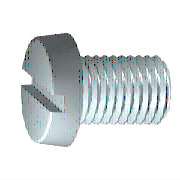
# Autodesk Inventor part: ISO 1207 - M4 x 14
Saved by Autodesk Inventor 2025.2 (Build 292293000, 293)
## iProperties
Created: 2024-01-20
Part Number: ISO 1207 - M4 x 14
Material: Stainless Steel, 440C
Description: Slotted cheese head screws - Product grade A
Document SubType Name: Modeling
Standard: ISO 1207
Designer: Kacper Mik
Standard Revision: Third edition 2011-08-01
Standards Organization: ISO
Language: en-US
Size Designation: M4 x 14
Categories: <MemberInstance><Categories><Category DisplayName="Fasteners" InternalName="e4da775c-781d-43d5-af7c-5136215cf5a6" Mnemonic="FSTN"><Category DisplayName="Bolts" InternalName="536e6df0-f778-49ac-b2f2-25c71d2aa0b2" Mnemonic="SCRW"><CategoryParameter DisplayName="Nominal Diameter Designation" InternalName="03caf894-eafd-4c09-a035-916ac084b87b" Mnemonic="nomdiadesig"/><CategoryParameter DisplayName="Nominal Length" InternalName="238ecbaf-3e6c-45dd-aa95-4068c8e0fd02" Mnemonic="nomlen"/><CategoryParameter DisplayName="Thread Designation" InternalName="586d5e89-370a-4089-914f-0110033585c7" Mnemonic="thrdesign"/><CategoryParameter DisplayName="Thread Series Designation" InternalName="87c5849c-b3a5-4c3e-9c9b-2feecef9be86" Mnemonic="thrserdsgn"/><CategoryParameter DisplayName="Nominal Diameter" InternalName="8bbe3f8e-44cf-40a9-a251-3a6edc8168d6" Mnemonic="nomdia"/><CategoryParameter DisplayName="Thread Type" InternalName="b4bbb7bc-d6aa-4c9f-a9a9-4152b9f6fe49" Mnemonic="thrtype"/><CategoryParameter DisplayName="Thread Pitch" InternalName="bb82302e-82d8-4176-8fc1-c5d7bb17d5ad" Mnemonic="pitch1"/><CategoryParameter DisplayName="Threads per Unit" InternalName="bdc6e7d2-ffd0-4d9c-a173-16b95ebb912d" Mnemonic="thrperunit1"/><CategoryParameter DisplayName="Thread Class" InternalName="ebc0d23b-2cc6-4d2a-b376-d52aae53bab6" Mnemonic="thrclss"/><Category DisplayName="Socket Head" InternalName="55e06bf3-7e58-486c-bbdc-745fcc60664d" Mnemonic="CLSCRW"><CategoryParameter DisplayName="Shank Diameter" InternalName="179dbae3-102f-48bb-85fe-1e3ecd34f7cc" Mnemonic="grpdia"/><CategoryParameter DisplayName="Thread Length" InternalName="3268731d-5f9a-4750-8b01-4a959c46fbf2" Mnemonic="thrlen"/><CategoryParameter DisplayName="Head Diameter" InternalName="46177176-dbdd-4a1b-aefd-4c60c45016af" Mnemonic="headdia"/><CategoryParameter DisplayName="Grip Length" InternalName="52eab69f-422f-4795-9995-175a1b827e67" Mnemonic="grplen"/><CategoryParameter DisplayName="Type" InternalName="59a7e495-7a0c-4a5c-bdfd-c090c5f6e2db" Mnemonic="type"/><CategoryParameter DisplayName="Head Height" InternalName="99c92c4c-4a02-4ebe-9e64-948fb169e19e" Mnemonic="headh"/></Category></Category></Category><Category DisplayName="DataType" InternalName="23b78d0f-2648-40c6-8793-ca6db495c9e8" Mnemonic="DATATYPE"><CategoryParameter DisplayName="DisplayName" InternalName="05415f3d-3907-474b-a020-eb9d644f4cf3" Mnemonic="DISPLAYNAME"/><CategoryParameter DisplayName="Standard" InternalName="0c0a119c-1e12-4c84-803f-101930972f5e" Mnemonic="STANDARD"/><CategoryParameter DisplayName="Description" InternalName="13903e3d-64b1-4950-80da-f627842ea37f" Mnemonic="DESCRIPTION"/><CategoryParameter DisplayName="Designation" InternalName="2675968c-4ce5-49e0-a4f5-552d29089031" Mnemonic="DESIGNATION"/><CategoryParameter DisplayName="Default Row" InternalName="2af9ec52-faaa-4026-b378-f9fa4afca842" Mnemonic="DEFAULTROW"/><CategoryParameter DisplayName="Folder Name" InternalName="3f06958e-8713-4116-9be7-ed6184ecc97b" Mnemonic="FOLDERNAME"/><CategoryParameter DisplayName="Revision Guid" InternalName="45a75005-10b1-4dfc-8d6d-dfe629f0b93c" Mnemonic="REVISIONGUID"/><CategoryParameter DisplayName="FileName" InternalName="8b46a4cc-9585-4fed-90c3-899f57e09a73" Mnemonic="FILENAME"/><CategoryParameter DisplayName="StdsOrg" InternalName="8f5914e1-4693-403f-8ab5-d37768198c9d" Mnemonic="STDSORG"/><CategoryParameter DisplayName="Family Version" InternalName="914462f6-6e19-4b14-ba84-155b9680b1d0" Mnemonic="FAMILYREVISION"/><CategoryParameter DisplayName="Standard Revision" InternalName="91d5a463-65c2-4fde-b823-3b7fea5e8e17" Mnemonic="STANDARDREVISION"/><CategoryParameter DisplayName="Member Revision" InternalName="a65d44b9-392f-4f4f-857b-e4b3d54996fe" Mnemonic="MEMBERREVISION"/><CategoryParameter DisplayName="ClipFormat" InternalName="bc51e27b-3422-4e78-93ef-cec197ddf230" Mnemonic="CLIPFORMAT"/><CategoryParameter DisplayName="Manufacturer" InternalName="cd6c7a72-a28a-4e50-99a9-2c7f4e13e5ad" Mnemonic="MANUFACTURER"/><CategoryParameter DisplayName="InternalName" InternalName="cf1d0246-76d9-4b4a-8305-fa0409afb5c1" Mnemonic="INTERNALNAME"/><CategoryParameter DisplayName="IsMetric" InternalName="e2385c5b-1ea4-4823-96a8-8de651266ec3" Mnemonic="ISMETRIC"/><Category DisplayName="Part" InternalName="c0e0b642-3bcb-4cc8-9e80-f96d35c4afa4" Mnemonic="PART"><CategoryParameter DisplayName="Part Number" InternalName="016b6077-bfbe-49bd-92c9-d8d59c39c941" Mnemonic="PARTNUMBER"/><CategoryParameter DisplayName="Stock Number" InternalName="4dba7c1c-e26c-444e-836c-b08b433409a8" Mnemonic="STOCKNUMBER"/><CategoryParameter DisplayName="Material Key" InternalName="5c9a8adb-dd2b-4535-b97f-0a94a95fe41f" Mnemonic="MATERIALKEY"/><CategoryParameter DisplayName="Material" InternalName="818a152a-d3c3-49ca-80ee-df7d91421b8e" Mnemonic="MATERIAL"/></Category></Category><Category DisplayName="Legacy Map DA" InternalName="924fff40-ddd0-4eff-ad42-30e3774ef79e" Mnemonic="LEGACYMAPDA"><CategoryParameter DisplayName="DACookie" InternalName="316934ee-8fe1-4c7a-9c36-f2d79e1add1a" Mnemonic="DACOOKIE"/></Category><Category DisplayName="LegacyMap" InternalName="cd87c42b-3e48-431e-b5c0-1cbeb14dfe77" Mnemonic="LEGACYMAP"><CategoryParameter DisplayName="unique DA member ID" InternalName="0918ad47-427f-4fed-ae26-24c81c58f590" Mnemonic="DACOOKIE"/><CategoryParameter DisplayName="Merge11 ID" InternalName="0ee8fb18-e2ed-4f39-96f6-1f4b5f50aa71" Mnemonic="MERGE11"/><CategoryParameter DisplayName="unique CC member ID" InternalName="5193edd4-b2b0-4ab4-9d54-de900eee34e0" Mnemonic="CCCOOKIE"/><CategoryParameter DisplayName="Split ID" InternalName="72b5c83c-be7f-45c4-ae51-9160ea6deb26" Mnemonic="SPLIT"/><CategoryParameter DisplayName="MemberID" InternalName="8e5e0294-fc51-4c8f-b3d7-003dc5ed94f6" Mnemonic="MEMBERID"/><CategoryParameter DisplayName="CatalogName" InternalName="d99d1e27-aa94-4de2-af4c-c348882a6f4f" Mnemonic="CATALOGNAME"/><CategoryParameter DisplayName="FamilyNumber" InternalName="e705e1f4-09cb-413e-91f9-551b4188271e" Mnemonic="FAMILYNUMBER"/></Category></Categories><FamilyTemplate Id="si0146"><FamilyTemplateParameters><FamilyTemplateParameter ObjectType="kUserParameterObject" ValueType="xs:double" Id="1" ObjectReferenceKey="GUL"/><FamilyTemplateParameter ObjectType="kUserParameterObject" ValueType="xs:double" Id="2" ObjectReferenceKey="SPD"/><FamilyTemplateParameter ObjectType="kUserParameterObject" ValueType="xs:double" Id="3" ObjectReferenceKey="NLG"/><FamilyTemplateParameter ObjectType="kUserParameterObject" ValueType="xs:double" Id="4" ObjectReferenceKey="KOD"/><FamilyTemplateParameter ObjectType="kUserParameterObject" ValueType="xs:double" Id="5" ObjectReferenceKey="SBR"/><FamilyTemplateParameter ObjectType="kUserParameterObject" ValueType="xs:double" Id="6" ObjectReferenceKey="PTC"/><FamilyTemplateParameter ObjectType="kUserParameterObject" ValueType="xs:double" Id="7" ObjectReferenceKey="GEL"/><FamilyTemplateParameter ObjectType="kUserParameterObject" ValueType="xs:double" Id="8" ObjectReferenceKey="THREADDIA"/><FamilyTemplateParameter ObjectType="kUserParameterObject" ValueType="xs:double" Id="9" ObjectReferenceKey="TOA"/><FamilyTemplateParameter ObjectType="kUserParameterObject" ValueType="xs:double" Id="10" ObjectReferenceKey="BDM"/><FamilyTemplateParameter ObjectType="kUserParameterObject" ValueType="xs:double" Id="11" ObjectReferenceKey="RR"/><FamilyTemplateParameter ObjectType="kUserParameterObject" ValueType="xs:double" Id="12" ObjectReferenceKey="STI"/><FamilyTemplateParameter ObjectType="kUserParameterObject" ValueType="xs:double" Id="13" ObjectReferenceKey="TPU"/><FamilyTemplateParameter ObjectType="kUserParameterObject" ValueType="xs:double" Id="14" ObjectReferenceKey="KOH"/><FamilyTemplateParameter ObjectType="kUserParameterObject" ValueType="xs:double" Id="15" ObjectReferenceKey="NND"/><FamilyTemplateParameter ObjectType="kUserParameterObject" ValueType="xs:double" Id="16" ObjectReferenceKey="GD"/><FamilyTemplateParameter ObjectType="kUserParameterObject" ValueType="xs:double" Id="17" ObjectReferenceKey="GAL"/><FamilyTemplateParameter ObjectType="kUserParameterObject" ValueType="xs:double" Id="18" ObjectReferenceKey="KEWI"/><FamilyTemplateParameter ObjectType="kUserParameterObject" ValueType="xs:double" Id="19" ObjectReferenceKey="GD1"/><FamilyTemplateParameter ObjectType="kPropertyObject" ValueType="xs:string" Id="100" ObjectReferenceKey="{32853F0F-3444-11d1-9E93-0060B03C1CA6}" SubObjectId="52"/><FamilyTemplateParameter ObjectType="kPropertyObject" ValueType="xs:string" Id="105" ObjectReferenceKey="{32853F0F-3444-11d1-9E93-0060B03C1CA6}" SubObjectId="5"/><FamilyTemplateParameter ObjectType="kPartComponentDefinitionObject" ValueType="xs:string" Id="110" SubObjectId="Material"/><FamilyTemplateParameter ObjectType="kThreadFeatureObject" ValueType="xs:structure" Id="300" ObjectReferenceKey="100200001000000000100000000000008000000000000000" SubObjectId="ThreadInfo"><FamilyTemplateParameter ObjectType="" ValueType="xs:string" Id="301" SubObjectId="ThreadDesignation"/><FamilyTemplateParameter ObjectType="" ValueType="xs:string" Id="302" SubObjectId="ThreadType"/><FamilyTemplateParameter ObjectType="" ValueType="xs:string" Id="303" SubObjectId="ThreadClass"/></FamilyTemplateParameter></FamilyTemplateParameters></FamilyTemplate><CategoryParameterMap><ParamToTemplateMap><ParamToTemplate CategoryParameter="//CategoryParameter[@InternalName='05415f3d-3907-474b-a020-eb9d644f4cf3']" ConstantValue="ISO 1207"/><ParamToTemplate CategoryParameter="//CategoryParameter[@InternalName='cf1d0246-76d9-4b4a-8305-fa0409afb5c1']" ConstantValue="e74c2f17-23da-4af6-900a-1ad8a84727ec"/><ParamToTemplate CategoryParameter="//CategoryParameter[@InternalName='3f06958e-8713-4116-9be7-ed6184ecc97b']" ConstantValue="ISO 1207(2)"/><ParamToTemplate CategoryParameter="//CategoryParameter[@InternalName='914462f6-6e19-4b14-ba84-155b9680b1d0']" ConstantValue="10"/><ParamToTemplate CategoryParameter="//CategoryParameter[@InternalName='bc51e27b-3422-4e78-93ef-cec197ddf230']" ConstantValue="CF_INVENTOR.STDPARTS"/><ParamToTemplate CategoryParameter="//CategoryParameter[@InternalName='e2385c5b-1ea4-4823-96a8-8de651266ec3']" ConstantValue="true"/><ParamToTemplate CategoryParameter="//CategoryParameter[@InternalName='13903e3d-64b1-4950-80da-f627842ea37f']" ConstantValue="Slotted cheese head screws - Product grade A"/><ParamToTemplate CategoryParameter="//CategoryParameter[@InternalName='8f5914e1-4693-403f-8ab5-d37768198c9d']" ConstantValue="ISO"/><ParamToTemplate CategoryParameter="//CategoryParameter[@InternalName='0c0a119c-1e12-4c84-803f-101930972f5e']" ConstantValue="ISO 1207"/><ParamToTemplate CategoryParameter="//CategoryParameter[@InternalName='cd6c7a72-a28a-4e50-99a9-2c7f4e13e5ad']" TemplateParameter="104"/><ParamToTemplate CategoryParameter="//CategoryParameter[@InternalName='91d5a463-65c2-4fde-b823-3b7fea5e8e17']" ConstantValue="Third edition 2011-08-01"/><ParamToTemplate CategoryParameter="//CategoryParameter[@InternalName='45a75005-10b1-4dfc-8d6d-dfe629f0b93c']" ConstantValue="7b1522c6-d84a-47e3-bf11-e7369115629e"/><ParamToTemplate CategoryParameter="//CategoryParameter[@InternalName='2af9ec52-faaa-4026-b378-f9fa4afca842']" ConstantValue="10"/><ParamToTemplate CategoryParameter="//CategoryParameter[@InternalName='d99d1e27-aa94-4de2-af4c-c348882a6f4f']" ConstantValue="ISO"/><ParamToTemplate CategoryParameter="//CategoryParameter[@InternalName='e705e1f4-09cb-413e-91f9-551b4188271e']" ConstantValue="12"/><ParamToTemplate CategoryParameter="//CategoryParameter[@InternalName='8b46a4cc-9585-4fed-90c3-899f57e09a73']" ConstantValue="ISO 1207 - M4 x 14"/><ParamToTemplate CategoryParameter="//CategoryParameter[@InternalName='a65d44b9-392f-4f4f-857b-e4b3d54996fe']" ConstantValue="5B6D940F-5202-4BE6-98E7-197EC5CCA440"/><ParamToTemplate CategoryParameter="//CategoryParameter[@InternalName='52eab69f-422f-4795-9995-175a1b827e67']" ConstantValue="1,4"/><ParamToTemplate CategoryParameter="//CategoryParameter[@InternalName='ebc0d23b-2cc6-4d2a-b376-d52aae53bab6']" ConstantValue="6g"/><ParamToTemplate CategoryParameter="//CategoryParameter[@InternalName='03caf894-eafd-4c09-a035-916ac084b87b']" ConstantValue="M4"/><ParamToTemplate CategoryParameter="//CategoryParameter[@InternalName='b4bbb7bc-d6aa-4c9f-a9a9-4152b9f6fe49']" ConstantValue="ISO Metric profile"/><ParamToTemplate CategoryParameter="//CategoryParameter[@InternalName='8e5e0294-fc51-4c8f-b3d7-003dc5ed94f6']" ConstantValue="590"/><ParamToTemplate CategoryParameter="//CategoryParameter[@InternalName='316934ee-8fe1-4c7a-9c36-f2d79e1add1a']" ConstantValue="*Iso~I1207~M4x14~14*"/><ParamToTemplate CategoryParameter="//CategoryParameter[@InternalName='179dbae3-102f-48bb-85fe-1e3ecd34f7cc']" TemplateParameter="10"/><ParamToTemplate CategoryParameter="//CategoryParameter[@InternalName='2675968c-4ce5-49e0-a4f5-552d29089031']" TemplateParameter="100"/><ParamToTemplate CategoryParameter="//CategoryParameter[@InternalName='3268731d-5f9a-4750-8b01-4a959c46fbf2']" TemplateParameter="7"/><ParamToTemplate CategoryParameter="//CategoryParameter[@InternalName='46177176-dbdd-4a1b-aefd-4c60c45016af']" TemplateParameter="4"/><ParamToTemplate CategoryParameter="//CategoryParameter[@InternalName='99c92c4c-4a02-4ebe-9e64-948fb169e19e']" TemplateParameter="14"/><ParamToTemplate CategoryParameter="//CategoryParameter[@InternalName='818a152a-d3c3-49ca-80ee-df7d91421b8e']" TemplateParameter="110"/><ParamToTemplate CategoryParameter="//CategoryParameter[@InternalName='238ecbaf-3e6c-45dd-aa95-4068c8e0fd02']" TemplateParameter="3"/><ParamToTemplate CategoryParameter="//CategoryParameter[@InternalName='8bbe3f8e-44cf-40a9-a251-3a6edc8168d6']" TemplateParameter="15"/><ParamToTemplate CategoryParameter="//CategoryParameter[@InternalName='016b6077-bfbe-49bd-92c9-d8d59c39c941']" TemplateParameter="105"/><ParamToTemplate CategoryParameter="//CategoryParameter[@InternalName='bb82302e-82d8-4176-8fc1-c5d7bb17d5ad']" TemplateParameter="6"/><ParamToTemplate CategoryParameter="//CategoryParameter[@InternalName='586d5e89-370a-4089-914f-0110033585c7']" TemplateParameter="301"/><ParamToTemplate CategoryParameter="//CategoryParameter[@InternalName='bdc6e7d2-ffd0-4d9c-a173-16b95ebb912d']" TemplateParameter="13"/></ParamToTemplateMap></CategoryParameterMap></MemberInstance>
Density: 7.75 g/cm^3
Appearance: Semi-Polished
IsCustomPart: 0
Author: Kacper Mik
Autodesk Inventor part; units mm, degrees
ref_plane "YZ Plane" through (0, 0, 0) normal (1, 0, 0) x (0, 1, 0)
ref_plane "XZ Plane" through (0, 0, 0) normal (0, 1, 0) x (-1, 0, 0)
sketch "Sketch1" plane through (0, 0, 0) normal (0, 0, 1) x (1, 0, 0)
  line L0 (-2.6, 0) -> (14, 0)
  line L1 (14, 0) -> (14, 2)
  line L2 (14, 2) -> (1.4, 2)
  line L3 (1.4, 2) -> (0.9705, 1.7853)
  line L4 (0.9705, 1.7853) -> (0, 1.7853)
  line L5 (0, 1.7853) -> (0, 3.5)
  line L6 (-5.92, 0) -> (17.32, 0) projected
  line L7 (0, -0.7) -> (0, 4.2) projected
  line L8 (-2.6, 0) -> (-2.6, 3.2725)
  line L9 (0, 3.5) -> (-2.6, 3.2725)
  line L10 (1.4, 2) -> (0, 2) construction
  dimension "d0" = 14
  dimension "d1" = 12.6
  dimension "d2" = 0.4295
  dimension "d3" = 2.6
  dimension "d4" = 4
  dimension "d5" = 3.5705
  dimension "d9" = 7
  dimension "d10" = 5
  constraints: 18 end point, 4 parallel, 2 collinear, 2 perpendicular, 1 horizontal, 1 point on line
  measures "d0" distance between parallel lines of L1 L5
  measures "d1" distance from line of L2.end L1
  measures "d2" horizontal distance of L3.end L2.end
  measures "d3" distance from line of L0.start L5
  measures "d4" diameter of L2 L0
  measures "d5" diameter of L4 L0
  measures "d9" diameter of L5.end L0
  measures "d10" angle of L9 L0
revolve "Body" add sketch "Sketch1" angle 360 about axis through (-2.6, 0, 0) along (1, 0, 0)
sketch "Sketch2" plane through (-2.6, 0, 0) normal (-1, 0, 0) x (0, 0, 1)
  circle A0 centre (0, 0) radius 3.5 projected
  line L0 (0, 0) -> (0, 3.2725) projected
  line L1 (-3.5, 0.6) -> (3.5, 0.6)
  line L2 (3.5, 0.6) -> (3.5, -0.6)
  line L3 (3.5, -0.6) -> (-3.5, -0.6)
  line L4 (-3.5, -0.6) -> (-3.5, 0.6)
  line L5 (-3.5, 0) -> (3.5, 0) construction
  line L6 (0, 0.6) -> (0, -0.6) construction
  dimension "d11" = 1.2
  dimension "d12" = 7
  constraints: 12 end point, 5 midpoint, 2 parallel, 1 collinear, 1 horizontal, 1 perpendicular
  measures "d11" distance of L3.end L1.start
  measures "d12" distance of L1.start L1.end
fillet "Fillet1" radius 0.2 1 edges at (-2.6, -3.2725, 0)
extrude "Slot" cut sketch "Sketch2" against normal blind 1.1 contours A0 L3 L1 | L2 L3 A0 | A0 L1 L2 | A0 L4 L1 | L3 L4 A0
thread "Thread" size "M4x0.7" class "6g" standard "ISO Metric profile" length 12.6
chamfer "Chamfer1" distance 0.4294 distance2 0.4295 1 edges at (14, -2, 0) measured on face at (14, 0.6473, -0.1595)
ref_plane "Work Plane1" through (30.1625, 0, 0) normal (0, 0, -1) x (1, 0, 0)
equation "\"d11\" = SBR"
equation "\"d12\" = KOD"
equation "\"d19\" = STI"
equation "\"d14\" = RR"
equation "\"d15\" = GEL"
equation "\"d17\" = -0.5 * SPD + 0.5 * GD"
equation "\"d0\" = NLG"
equation "\"d1\" = GEL"
equation "\"d3\" = KOH"
equation "\"d4\" = GD"
equation "\"d5\" = BDM"
equation "\"d9\" = KOD"
equation "\"d10\" = KEWI"
equation "\"GD\" = NND"
equation "\"NLG\" = 14"
equation "\"GEL\" = 12.6"
equation "\"KOD\" = 7"
equation "\"KOH\" = 2.6"
equation "\"GAL\" = 0.61345 * PTC"
equation "\"SPD\" = NND - 1.2269 * PTC"
equation "\"BDM\" = 3.5705"
equation "\"GUL\" = 0.61345 * PTC"
equation "\"RR\" = 0.2"
equation "\"SBR\" = 1.2"
equation "\"STI\" = 1.1"
equation "\"KEWI\" = 5deg"
equation "\"PTC\" = 0.7"
equation "\"THREADDIA\" = 4"
equation "\"TOA\" = 30deg"
equation "\"NND\" = 4"
equation "\"GD1\" = THREADDIA - 1.2269 * PTC"
body "Solid1"
